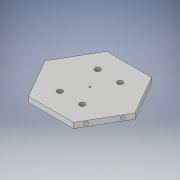
# Autodesk Inventor part: Hex_Servo_Top
Saved by Autodesk Inventor 2019.4 (Build 234330000, 330)
## iProperties
Created: 2019-09-26
Part Number: Hex_Servo_Top
Material: Generic
Document SubType Name: Modeling
Designer: Jorian Bruslind
Density: 1 g/cm^3
Appearance: Default
Author: Jorian Bruslind
Autodesk Inventor part; units mm, degrees
ref_plane "YZ Plane" through (0, 0, 0) normal (1, 0, 0) x (0, 1, 0)
ref_plane "XZ Plane" through (0, 0, 0) normal (0, 1, 0) x (-1, 0, 0)
ref_plane "XY Plane" through (0, 0, 0) normal (0, 0, 1) x (1, 0, 0)
sketch "Sketch1" plane through (0, 0, 0) normal (0, 1, 0) x (-1, 0, 0)
  line L0 (25, 0) -> (12.5, -21.6506)
  line L1 (12.5, -21.6506) -> (-12.5, -21.6506)
  line L2 (-12.5, -21.6506) -> (-25, 0)
  line L3 (-25, 0) -> (-12.5, 21.6506)
  line L4 (-12.5, 21.6506) -> (12.5, 21.6506)
  line L5 (12.5, 21.6506) -> (25, 0)
  point P0 (0, 0)
  point P1 (0, 0)
  dimension "d0" = 25
  dimension "d17" = 21.6506
  constraints: 12 end point, 1 coincident, 13 other
  measures "d0" distance of L0.end L1.end
  measures "d17" vertical distance of L4.end L0.start
extrude "Extrusion1" add sketch "Sketch1" along normal blind 3
sketch "Sketch2" plane through (25, 0, 0) normal (0.8660254, 0, 0.5) x (0.5, 0, -0.8660254)
  line L0 (0, 0) -> (0, 3) projected
  line L1 (0, 1.5) -> (-5, 1.5)
  line L2 (-25, 0) -> (-25, 3) projected
  line L3 (-25, 1.5) -> (-20, 1.5)
  circle A0 centre (-20, 1.5) radius 1
  circle A1 centre (-5, 1.5) radius 1
  point P0 (-12.5, 0)
  dimension "d4" = 5
  dimension "d5" = 5
  dimension "d6" = 2
  dimension "d7" = 2
  constraints: 4 end point, 2 centre point, 2 coincident, 2 horizontal, 2 midpoint
  measures "d4" distance of L1.start L1.end
  measures "d5" distance of L3.start L3.end
  measures "d6" diameter of A0
  measures "d7" diameter of A1
extrude "Extrusion2" cut sketch "Sketch2" against normal blind 5
sketch "Sketch3" plane through (0, 3, 0) normal (0, 1, 0) x (1, 0, 0)
  circle A0 centre (0, 0) radius 0.5
  dimension "d10" = 1
  constraints: 1 centre point, 1 coincident
  measures "d10" diameter of A0
extrude "Extrusion3" cut sketch "Sketch3" against normal blind 5
pattern_circular "Circular Pattern1" count 3 over 360 about axis through (0, 3, 0) along (0, -1, 0) of "Extrusion2"
sketch "Sketch4" plane through (0, 3, 0) normal (0, 1, 0) x (1, 0, 0)
  line L0 (0, 0) -> (0, 10.5)
  line L1 (0, 10.5) -> (-6.25, 10.5)
  circle A0 centre (-6.25, 10.5) radius 1.5
  circle A1 centre (6.25, 10.5) radius 1.5
  circle A2 centre (-6.25, -10.5) radius 1.5
  circle A3 centre (6.25, -10.5) radius 1.5
  dimension "d18" = 10.5
  dimension "d19" = 6.25
  dimension "d20" = 3
  dimension "d23" = 12.5
  dimension "d26" = 21
  constraints: 4 centre point, 4 end point, 2 vertical, 1 coincident, 1 horizontal, 1 perpendicular, 6 other
  measures "d18" distance of L0.start L0.end
  measures "d19" distance of L0.end L1.end
  measures "d20" diameter of A0
  measures "d23" distance of A0.centre A1.centre
  measures "d26" distance of A0.centre A2.centre
extrude "Extrusion4" cut sketch "Sketch4" against normal blind 5
body "Solid1"
